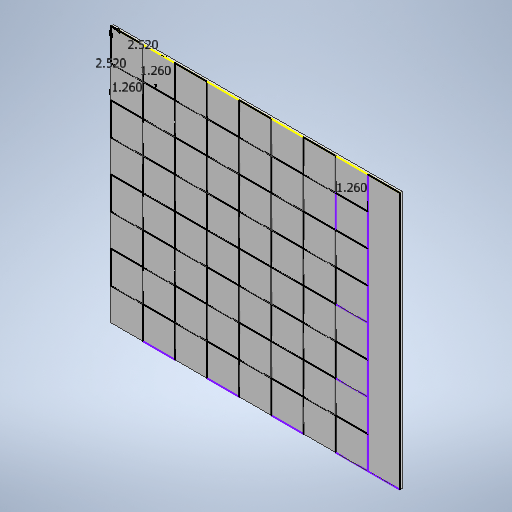
# Autodesk Inventor part: Floor
Saved by Autodesk Inventor 2025.2 (Build 292293000, 293)
## iProperties
Created: 2025-04-23
Part Number: Floor
Material: Generic
Document SubType Name: Modeling
Designer: powel
Density: 1 g/cm^3
Appearance: Default
Author: powel
Autodesk Inventor part; units mm, degrees
ref_plane "YZ Plane" through (0, 0, 0) normal (1, 0, 0) x (0, 1, 0)
ref_plane "XZ Plane" through (0, 0, 0) normal (0, 1, 0) x (-1, 0, 0)
ref_plane "XY Plane" through (0, 0, 0) normal (0, 0, 1) x (1, 0, 0)
sketch "Sketch1" plane through (0, 0, 0) normal (0, 0, 1) x (1, 0, 0)
  line L0 (0, 0) -> (-288, 0)
  line L1 (-288, 0) -> (-288, -256)
  line L2 (-288, -256) -> (0, -256)
  line L3 (0, -256) -> (0, 0)
  dimension "d0" = 288
  dimension "d1" = 256
  constraints: 8 end point, 2 parallel, 1 horizontal, 1 perpendicular
  measures "d0" distance of L2.end L1.end
  measures "d1" distance of L1.end L0.end
extrude "Extrusion1" add sketch "Sketch1" along normal blind 2.54
sketch "Sketch2" plane through (0, 0, 2.54) normal (0, 0, 1) x (1, 0, 0)
  line L0 (-288, 0) -> (-256, 0)
  line L1 (-256, 0) -> (-256, -32)
  line L2 (-256, -32) -> (-288, -32)
  line L3 (-288, -32) -> (-288, 0)
  line L4 (-224, 0) -> (-192, 0)
  line L5 (-192, 0) -> (-192, -32)
  line L6 (-192, -32) -> (-224, -32)
  line L7 (-224, -32) -> (-224, 0)
  line L8 (-160, 0) -> (-128, 0)
  line L9 (-128, 0) -> (-128, -32)
  line L10 (-128, -32) -> (-160, -32)
  line L11 (-160, -32) -> (-160, 0)
  line L12 (-96, 0) -> (-64, 0)
  line L13 (-64, 0) -> (-64, -32)
  line L14 (-64, -32) -> (-96, -32)
  line L15 (-96, -32) -> (-96, 0)
  line L16 (-288, -64) -> (-256, -64)
  line L17 (-256, -64) -> (-256, -96)
  line L18 (-256, -96) -> (-288, -96)
  line L19 (-288, -96) -> (-288, -64)
  line L20 (-224, -64) -> (-192, -64)
  line L21 (-192, -64) -> (-192, -96)
  line L22 (-192, -96) -> (-224, -96)
  line L23 (-224, -96) -> (-224, -64)
  line L24 (-160, -64) -> (-128, -64)
  line L25 (-128, -64) -> (-128, -96)
  line L26 (-128, -96) -> (-160, -96)
  line L27 (-160, -96) -> (-160, -64)
  line L28 (-96, -64) -> (-64, -64)
  line L29 (-64, -64) -> (-64, -96)
  line L30 (-64, -96) -> (-96, -96)
  line L31 (-96, -96) -> (-96, -64)
  line L32 (-288, -128) -> (-256, -128)
  line L33 (-256, -128) -> (-256, -160)
  line L34 (-256, -160) -> (-288, -160)
  line L35 (-288, -160) -> (-288, -128)
  line L36 (-224, -128) -> (-192, -128)
  line L37 (-192, -128) -> (-192, -160)
  line L38 (-192, -160) -> (-224, -160)
  line L39 (-224, -160) -> (-224, -128)
  line L40 (-160, -128) -> (-128, -128)
  line L41 (-128, -128) -> (-128, -160)
  line L42 (-128, -160) -> (-160, -160)
  line L43 (-160, -160) -> (-160, -128)
  line L44 (-96, -128) -> (-64, -128)
  line L45 (-64, -128) -> (-64, -160)
  line L46 (-64, -160) -> (-96, -160)
  line L47 (-96, -160) -> (-96, -128)
  line L48 (-288, -192) -> (-256, -192)
  line L49 (-256, -192) -> (-256, -224)
  line L50 (-256, -224) -> (-288, -224)
  line L51 (-288, -224) -> (-288, -192)
  line L52 (-224, -192) -> (-192, -192)
  line L53 (-192, -192) -> (-192, -224)
  line L54 (-192, -224) -> (-224, -224)
  line L55 (-224, -224) -> (-224, -192)
  line L56 (-160, -192) -> (-128, -192)
  line L57 (-128, -192) -> (-128, -224)
  line L58 (-128, -224) -> (-160, -224)
  line L59 (-160, -224) -> (-160, -192)
  line L60 (-96, -192) -> (-64, -192)
  line L61 (-64, -192) -> (-64, -224)
  line L62 (-64, -224) -> (-96, -224)
  line L63 (-96, -224) -> (-96, -192)
  line L64 (-256, -64) -> (-224, -64)
  line L65 (-224, -64) -> (-224, -32)
  line L66 (-224, -32) -> (-256, -32)
  line L67 (-256, -32) -> (-256, -64)
  line L68 (-192, -64) -> (-160, -64)
  line L69 (-160, -64) -> (-160, -32)
  line L70 (-160, -32) -> (-192, -32)
  line L71 (-192, -32) -> (-192, -64)
  line L72 (-128, -64) -> (-96, -64)
  line L73 (-96, -64) -> (-96, -32)
  line L74 (-96, -32) -> (-128, -32)
  line L75 (-128, -32) -> (-128, -64)
  line L76 (-64, -64) -> (-32, -64)
  line L77 (-32, -32) -> (-64, -32)
  line L78 (-64, -32) -> (-64, -64)
  line L79 (-64, -96) -> (-32, -96)
  line L80 (-32, -96) -> (-32, -128)
  line L81 (-32, -128) -> (-64, -128)
  line L82 (-64, -128) -> (-64, -96)
  line L83 (-64, -160) -> (-32, -160)
  line L84 (-32, -160) -> (-32, -192)
  line L85 (-32, -192) -> (-64, -192)
  line L86 (-64, -192) -> (-64, -160)
  line L87 (-96, -192) -> (-128, -192)
  line L88 (-128, -192) -> (-128, -160)
  line L89 (-128, -160) -> (-96, -160)
  line L90 (-96, -160) -> (-96, -192)
  line L91 (-96, -128) -> (-128, -128)
  line L92 (-128, -128) -> (-128, -96)
  line L93 (-128, -96) -> (-96, -96)
  line L94 (-96, -96) -> (-96, -128)
  line L95 (-160, -128) -> (-192, -128)
  line L96 (-192, -128) -> (-192, -96)
  line L97 (-192, -96) -> (-160, -96)
  line L98 (-160, -96) -> (-160, -128)
  line L99 (-224, -128) -> (-256, -128)
  line L100 (-256, -128) -> (-256, -96)
  line L101 (-256, -96) -> (-224, -96)
  line L102 (-224, -96) -> (-224, -128)
  line L103 (-256, -160) -> (-224, -160)
  line L104 (-224, -160) -> (-224, -192)
  line L105 (-224, -192) -> (-256, -192)
  line L106 (-256, -192) -> (-256, -160)
  line L107 (-192, -160) -> (-160, -160)
  line L108 (-160, -160) -> (-160, -192)
  line L109 (-160, -192) -> (-192, -192)
  line L110 (-192, -192) -> (-192, -160)
  line L111 (-256, -224) -> (-224, -224)
  line L112 (-224, -224) -> (-224, -256)
  line L113 (-224, -256) -> (-256, -256)
  line L114 (-256, -256) -> (-256, -224)
  line L115 (-192, -224) -> (-160, -224)
  line L116 (-160, -224) -> (-160, -256)
  line L117 (-160, -256) -> (-192, -256)
  line L118 (-192, -256) -> (-192, -224)
  line L119 (-128, -224) -> (-96, -224)
  line L120 (-96, -224) -> (-96, -256)
  line L121 (-96, -256) -> (-128, -256)
  line L122 (-128, -256) -> (-128, -224)
  line L123 (-64, -224) -> (-32, -224)
  line L124 (-32, -224) -> (-32, -256)
  line L125 (-32, -256) -> (-64, -256)
  line L126 (-64, -256) -> (-64, -224)
  line L127 (-32, 0) -> (-32, -256)
  line L128 (0, 0) -> (-288, 0) projected
  line L129 (0, 0) -> (-32, 0)
  line L130 (-32, 0) -> (-32, -256)
  line L131 (-32, -256) -> (0, -256)
  line L132 (0, -256) -> (0, 0)
  dimension "d4" = 32
  dimension "d5" = 32
  dimension "d8" = 64
  dimension "d11" = 64
  dimension "d14" = 32
  constraints: 264 end point, 35 parallel, 19 horizontal, 17 perpendicular, 7 point on line, 3 collinear, 1 vertical, 119 other
  measures "d4" distance of L1.end L2.end
  measures "d5" distance of L0.end L1.end
  measures "d8" distance of L0.start L4.start
  measures "d11" distance of L0.start L16.start
  measures "d14" distance of L77.end L77.start
mark "Mark1"
body "Solid1"
